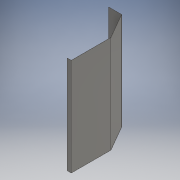
# Autodesk Inventor part: Cover Back
Saved by Autodesk Inventor 2018 (Build 220112000, 112)
## iProperties
Created: 2018-08-07
Part Number: Cover Back
Material: Stainless Steel
Document SubType Name: Modeling
Designer: P301319
Density: 8 g/cm^3
Appearance: Stainless - Brushed
Author: P301319
Autodesk Inventor part; units mm, degrees
ref_plane "YZ Plane" through (0, 0, 0) normal (1, 0, 0) x (0, 1, 0)
ref_plane "XZ Plane" through (0, 0, 0) normal (0, 1, 0) x (-1, 0, 0)
ref_plane "XY Plane" through (0, 0, 0) normal (0, 0, 1) x (1, 0, 0)
sketch "Sketch1" plane through (0, 0, 0) normal (0, 0, 1) x (1, 0, 0)
  line L0 (-340, 800) -> (-180, 800)
  line L1 (-180, 800) -> (0, 488.2309)
  line L2 (-180, 800) -> (122.4624, 800) construction
  line L3 (0, 0) -> (0, 488.2309)
  line L4 (0, 0) -> (-50, 0)
  line L5 (-50, 1.6) -> (-1.6, 1.6)
  line L6 (-1.6, 1.6) -> (-1.6, 487.8021)
  line L7 (-1.6, 487.8021) -> (-180.9238, 798.4)
  line L8 (-180.9238, 798.4) -> (-340, 798.4)
  line L9 (-50, 0) -> (-50, 1.6)
  line L10 (-340, 800) -> (-340, 798.4)
  dimension "d0" = 160
  dimension "d1" = 60
  dimension "d2" = 800
  dimension "d3" = 340
  dimension "d4" = 50
  dimension "d5" = 1.6
  constraints: 22 end point, 3 horizontal, 2 vertical, 1 perpendicular, 3 other
  measures "d0" distance of L0.start L0.end
  measures "d1" angle of L1 L2
  measures "d2" distance from line of L3.start L0
  measures "d3" horizontal distance of L3.start L0.start
  measures "d4" distance of L3.start L4.end
  measures "d5" distance between parallel lines of L1 L7
extrude "Extrusion1" add sketch "Sketch1" along normal blind 1200
body "Solid1"
